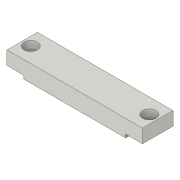
# Autodesk Inventor part: Anschlag
Saved by Autodesk Inventor 2018.3 (Build 223284000, 284)
## iProperties
Created: 2019-11-28
Material: Stahl, unlegiert
Document SubType Name: Modeling
Designer: bauermeisterdi
Density: 7.85 g/cm^3
Appearance: Stahl
Description: Anschlag
Werkstoff: S235JRC+C
Author: bauermeisterdi
Autodesk Inventor part; units mm, degrees
ref_plane "YZ Plane" through (0, 0, 0) normal (1, 0, 0) x (0, 1, 0)
ref_plane "XZ Plane" through (0, 0, 0) normal (0, 1, 0) x (-1, 0, 0)
ref_plane "XY Plane" through (0, 0, 0) normal (0, 0, 1) x (1, 0, 0)
sketch "Skizze_Grudnkörper" plane through (0, 0, 0) normal (0, 0, 1) x (1, 0, 0)
  line L0 (-56, 0) -> (56, 0) projected
  line L1 (0, -12.6) -> (0, 12.6) projected
  line L2 (40, -9) -> (-40, -9)
  line L3 (-40, -9) -> (-40, 9)
  line L4 (-40, 9) -> (40, 9)
  line L5 (40, 9) -> (40, -9)
  line L6 (40, -9) -> (-40, 9) construction
  line L7 (-40, -9) -> (40, 9) construction
  point P0 (0, 0)
  dimension "Länge" = 80
  dimension "Breite" = 18
  constraints: 12 end point, 2 midpoint, 2 parallel, 1 horizontal, 1 perpendicular
  measures "Länge" distance of L3.end L4.end
  measures "Breite" distance of L4.end L2.start
extrude "Grundkörper" add sketch "Skizze_Grudnkörper" along normal blind 10
sketch "Skizze_Senkbohrung" plane through (0, 0, 10) normal (0, 0, 1) x (1, 0, 0)
  line L0 (-56, 0) -> (56, 0) projected
  line L1 (0, -12.6) -> (0, 12.6) projected
  line L2 (-40, -9) -> (40, -9) projected
  line L3 (40, -9) -> (40, 9) projected
  line L4 (40, 9) -> (-40, 9) projected
  line L5 (-40, 9) -> (-40, -9) projected
  point P0 (0, 0)
  point P1 (-35, 0)
  point P2 (35, 0)
  dimension "d4" = 70
  constraints: 2 point on line, 1 symmetric about line
  measures "d4" distance of point (35, 0) point (-35, 0)
hole "Senkbohrung" at (-35, 0, 10) at (35, 0, 10) direction (0, 0, -1) diameter 4.5 end through all counterbore diameter 8 counterbore depth 4.6
sketch "Skizze_Ausnehmung" plane through (0, 0, 0) normal (0, 0, -1) x (-1, 0, 0)
  circle A0 centre (35, 0) radius 2.25 projected
  circle A1 centre (-35, 0) radius 2.25 projected
  line L0 (-40, -9) -> (40, -9) projected
  line L1 (40, -9) -> (40, 9) projected
  line L2 (40, 9) -> (-40, 9) projected
  line L3 (-40, 9) -> (-40, -9) projected
  line L4 (56, 0) -> (-56, 0) projected
  line L5 (0, -12.6) -> (0, 12.6) projected
  line L6 (40, 9) -> (-40, 9) projected
  line L7 (40, -9) -> (30, -9)
  line L8 (30, -9) -> (30, 9)
  line L9 (30, 9) -> (40, 9)
  line L10 (40, 9) -> (40, -9)
  line L11 (-40, 9) -> (-40, -9) projected
  line L12 (-40, -9) -> (-30, -9)
  line L13 (-30, -9) -> (-30, 9)
  line L14 (-30, 9) -> (-40, 9)
  line L15 (-40, 9) -> (-40, -9)
  point P0 (0, 0)
  dimension "d12" = 60
  constraints: 16 end point, 4 parallel, 2 horizontal, 2 perpendicular, 2 point on line, 1 other
  measures "d12" distance between parallel lines of L13 L8
extrude "Ausnehmung" cut sketch "Skizze_Ausnehmung" against normal blind 2 contours L4 L1 L0 L8 A0 | A0 L4 L8 L2 L1 | L13 L0 L3 L4 A1 | L4 A1 L3 L2 L13
